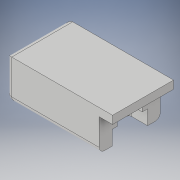
# Autodesk Inventor part: CajonSup
Saved by Autodesk Inventor 2019 (Build 230136000, 136)
## iProperties
Created: 2020-08-08
Part Number: CajonSup
Material: Generic
Document SubType Name: Modeling
Designer: Sergio
Density: 1 g/cm^3
Appearance: Default
Author: Sergio
Autodesk Inventor part; units mm, degrees
ref_plane "YZ Plane" through (0, 0, 0) normal (1, 0, 0) x (0, 1, 0)
ref_plane "XZ Plane" through (0, 0, 0) normal (0, 1, 0) x (-1, 0, 0)
ref_plane "XY Plane" through (0, 0, 0) normal (0, 0, 1) x (1, 0, 0)
sketch "Sketch1" plane through (0, 0, 0) normal (0, 1, 0) x (-1, 0, 0)
  line L0 (-3.75, -5.75) -> (3.75, -5.75) construction
  line L1 (3.75, -5.75) -> (3.75, 5.75) construction
  line L2 (3.75, 5.75) -> (-3.75, 5.75) construction
  line L3 (-3.75, 5.75) -> (-3.75, -5.75) construction
  line L4 (-3.75, -5.75) -> (3.75, 5.75) construction
  line L5 (3.75, -5.75) -> (-3.75, 5.75) construction
  line L6 (3.75, 5.75) -> (-16.25, 5.75)
  line L7 (-16.25, 5.75) -> (-16.25, -5.75)
  line L8 (-16.25, -5.75) -> (3.75, -5.75)
  line L9 (3.75, -5.75) -> (3.75, 5.75)
  point P0 (0, 0)
  dimension "d0" = 7.5
  dimension "d1" = 11.5
  dimension "d2" = 20
  constraints: 20 end point, 4 parallel, 2 horizontal, 2 midpoint, 2 perpendicular, 1 collinear
  measures "d0" distance of L2.end L1.end
  measures "d1" distance of L1.end L0.end
  measures "d2" distance of L8.end L7.end
extrude "Extrusion1" add sketch "Sketch1" along normal blind 7.5
sketch "Sketch2" plane through (16.25, 0, 5.75) normal (1, 0, 0) x (0, 0, -1)
  line L0 (3.4, 2.75) -> (8.1, 2.75)
  line L1 (8.1, 2.75) -> (8.1, 6)
  line L2 (8.1, 6) -> (3.4, 6)
  line L3 (3.4, 6) -> (3.4, 2.75)
  line L4 (0, 0) -> (0, 7.5) projected
  line L5 (11.5, 0) -> (11.5, 7.5) projected
  line L6 (0, 0) -> (11.5, 0) projected
  line L7 (0, 7.5) -> (11.5, 7.5) projected
  point P0 (5.75, 0)
  dimension "d5" = 3.4
  dimension "d6" = 3.4
  dimension "d7" = 2.75
  dimension "d8" = 1.5
  constraints: 8 end point, 2 parallel, 1 horizontal, 1 perpendicular
  measures "d5" distance between parallel lines of L4 L3
  measures "d6" distance between parallel lines of L5 L1
  measures "d7" distance between parallel lines of L6 L0
  measures "d8" distance between parallel lines of L7 L2
extrude "Extrusion2" cut sketch "Sketch2" against normal blind 18 contours L3 L2 L1 L0
sketch "Sketch3" plane through (16.25, 0, 5.75) normal (1, 0, 0) x (0, 0, -1)
  line L0 (2.4, 0) -> (9.1, 0)
  line L1 (9.1, 0) -> (9.1, 2.75)
  line L2 (9.1, 2.75) -> (2.4, 2.75)
  line L3 (2.4, 2.75) -> (2.4, 0)
  line L4 (8.1, 2.75) -> (3.4, 2.75) projected
  line L5 (0, 0) -> (11.5, 0) projected
  line L6 (3.4, 2.75) -> (3.4, 6) projected
  line L7 (8.1, 6) -> (8.1, 2.75) projected
  point P0 (5.75, 0)
  dimension "d12" = 1
  dimension "d14" = 1
  constraints: 8 end point, 2 collinear, 2 parallel, 1 horizontal, 1 perpendicular
  measures "d12" distance between parallel lines of L6 L3
  measures "d14" distance between parallel lines of L7 L1
extrude "Extrusion3" cut sketch "Sketch3" against normal blind 6
fillet "Fillet1" radius 0.5 5 edges at (10.25, 2.75, 0) (10.25, 1.375, 3.35) (10.25, 1.375, -3.35) (4.25, 2.75, -2.35) (4.25, 2.75, 2.35)
sketch "Sketch5" plane through (0, 0, 0) normal (0, -1, 0) x (1, 0, 0)
  line L0 (16.25, 5.75) -> (16.25, 3.35) projected
  line L1 (16.25, -5.75) -> (-3.75, -5.75) projected
  line L2 (16.25, 5.75) -> (13.75, 5.75)
  line L3 (13.75, 5.75) -> (13.75, -5.75)
  line L4 (13.75, -5.75) -> (16.25, -5.75)
  line L5 (16.25, -5.75) -> (16.25, 5.75)
  point P0 (0, 0)
  dimension "d18" = 2.5
  constraints: 8 end point, 2 parallel, 1 horizontal, 1 perpendicular, 1 point on line
  measures "d18" distance of L4.end L3.end
extrude "Extrusion4" cut sketch "Sketch5" against normal blind 6
fillet "Fillet2" radius 1 4 edges at (-3.75, 0, 0) (-3.75, 3.75, -5.75) (-3.75, 3.75, 5.75) (-3.75, 7.5, 0)
fillet "Fillet3" radius 1 4 edges at (-3.4571, 0.2929, -5.4571) (5.5, 0, -5.75) (-3.4571, 0.2929, 5.4571) (5.5, 0, 5.75)
body "Solid1"
